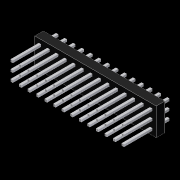
# Autodesk Inventor part: J25
Saved by Autodesk Inventor 2012 (Build 160160000, 160)
## iProperties
Company: Team 801
Created: 2009-08-01
Part Number: J25
Document SubType Name: Modeling
Designer: Jeffrey M
Density: 1 g/cm^3
Catalog Web Link: www.team801.org
Material: Default
Author: Jeffrey M
Autodesk Inventor part; units mm, degrees
ref_plane "YZ Plane" through (0, 0, 0) normal (1, 0, 0) x (0, 1, 0)
ref_plane "XZ Plane" through (0, 0, 0) normal (0, 1, 0) x (-1, 0, 0)
ref_plane "XY Plane" through (0, 0, 0) normal (0, 0, 1) x (1, 0, 0)
sketch "Sketch1" plane through (0, 0, 0) normal (0, 0, 1) x (1, 0, 0)
  line L0 (36.068, -8.128) -> (0, -8.128)
  line L1 (0, -8.128) -> (0, 0)
  line L2 (0, 0) -> (36.068, 0)
  line L3 (36.068, 0) -> (36.068, -8.128)
  line L4 (34.8615, -1.8415) -> (34.8615, -1.2065)
  line L5 (34.8615, -1.2065) -> (34.2265, -1.2065)
  line L6 (34.2265, -1.8415) -> (34.8615, -1.8415)
  line L7 (34.2265, -1.2065) -> (34.2265, -1.8415)
  line L8 (32.3215, -1.8415) -> (32.3215, -1.2065)
  line L9 (29.7815, -1.8415) -> (29.7815, -1.2065)
  line L10 (27.2415, -1.8415) -> (27.2415, -1.2065)
  line L11 (34.8615, -4.3815) -> (34.8615, -3.7465)
  line L12 (34.8615, -3.7465) -> (34.2265, -3.7465)
  line L13 (34.2265, -4.3815) -> (34.8615, -4.3815)
  line L14 (34.2265, -3.7465) -> (34.2265, -4.3815)
  line L15 (34.8615, -6.2865) -> (34.2265, -6.2865)
  line L16 (34.2265, -6.9215) -> (34.8615, -6.9215)
  line L17 (34.8615, -6.9215) -> (34.8615, -6.2865)
  line L18 (34.2265, -6.2865) -> (34.2265, -6.9215)
  dimension "d0" = 0
  dimension "d1" = 0.635
  dimension "d2" = 0.635
  dimension "d3" = 0.635
  dimension "d4" = 0.635
  dimension "d6" = 1.2065
  dimension "d7" = 1.2065
  constraints: 38 end point
  measures "d0" angle of L4 L8
  measures "d1" distance of L4.end L5.end
  measures "d2" distance of L5.end L7.end
  measures "d3" distance of L7.end L4.start
  measures "d4" distance of L4.start L4.end
  measures "d6" distance between parallel lines of L2 L5
  measures "d7" distance between parallel lines of L3 L4
extrude "Extrusion1" add sketch "Sketch1" against normal blind 2.54 contours L0 L1 L2 L3 | L6 L7 L5 L4 | L13 L14 L12 L11 | L17 L16 L18 L15
extrude "Extrusion2" add sketch "Sketch1" along normal blind 8.382 contours L6 L7 L5 L4
extrude "Extrusion3" add sketch "Sketch1" against normal blind 5.08 contours L6 L7 L5 L4
pattern_linear "Rectangular Pattern1" count 14 spacing 2.54 along (-1, 0, 0) count 3 spacing 2.54 along (0.000004, -1, 0) of "Extrusion2", "Extrusion3"
body "Solid1"
